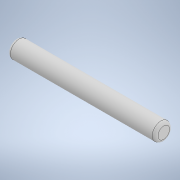
# Autodesk Inventor part: axle small
Saved by Autodesk Inventor 2022 (Build 260153070, 153G)
## iProperties
Created: 2021-07-02
Part Number: axle small
Material: Stainless Steel
Document SubType Name: Modeling
Designer: AKASH ARYAN
Density: 8 g/cm^3
Appearance: Semi-Polished
Author: AKASH ARYAN
Autodesk Inventor part; units mm, degrees
ref_plane "YZ Plane" through (0, 0, 0) normal (1, 0, 0) x (0, 1, 0)
ref_plane "XZ Plane" through (0, 0, 0) normal (0, 1, 0) x (-1, 0, 0)
ref_plane "XY Plane" through (0, 0, 0) normal (0, 0, 1) x (1, 0, 0)
sketch "Sketch1" plane through (0, 0, 0) normal (1, 0, 0) x (0, 1, 0)
  circle A0 centre (0, 0) radius 3
  dimension "d0" = 6
  constraints: 1 centre point, 1 coincident
  measures "d0" diameter of A0
extrude "Extrusion1" add sketch "Sketch1" along normal blind 50.8
fillet "Fillet1" radius 1 1 edges at (50.8, -3, 0)
fillet "Fillet2" radius 1 1 edges at (0, -3, 0)
body "Solid1"
